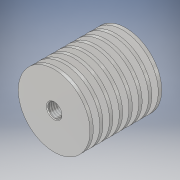
# Autodesk Inventor part: Cooling fin
Saved by Autodesk Inventor 2019 (Build 230136000, 136)
## iProperties
Created: 2018-11-13
Part Number: Cooling fin
Material: Aluminum 5005-H18
Document SubType Name: Modeling
Designer: LillaHunden
Density: 2.7 g/cm^3
Appearance: Aluminum - Polished
Author: LillaHunden
Autodesk Inventor part; units mm, degrees
ref_plane "YZ Plane" through (0, 0, 0) normal (1, 0, 0) x (0, 1, 0)
ref_plane "XZ Plane" through (0, 0, 0) normal (0, 1, 0) x (-1, 0, 0)
ref_plane "XY Plane" through (0, 0, 0) normal (0, 0, 1) x (1, 0, 0)
sketch "Sketch1" plane through (0, 0, 0) normal (0, 0, 1) x (1, 0, 0)
  circle A0 centre (0, 0) radius 12.5
  dimension "d0" = 25
  constraints: 1 centre point, 1 coincident
  measures "d0" diameter of A0
extrude "Extrusion1" add sketch "Sketch1" along normal blind 25
sketch "Sketch2" plane through (0, 0, 0) normal (1, 0, 0) x (0, 1, 0)
  line L0 (0, 0) -> (0, 24.8569) construction
  line L1 (12.5, 0) -> (12.5, 25) projected
  line L2 (12.5, 23.85) -> (4.58, 23.85)
  line L3 (4.58, 23.85) -> (4.58, 21.6)
  line L4 (4.58, 21.6) -> (12.5, 21.6)
  line L5 (12.5, 21.6) -> (12.5, 23.85)
  line L6 (12.5, 25) -> (-12.5, 25) projected
  line L7 (12.5, 20.45) -> (4.58, 20.45)
  line L8 (4.58, 20.45) -> (4.58, 18.2)
  line L9 (4.58, 18.2) -> (12.5, 18.2)
  line L10 (12.5, 18.2) -> (12.5, 20.45)
  line L11 (12.5, 17.05) -> (4.58, 17.05)
  line L12 (4.58, 17.05) -> (4.58, 14.8)
  line L13 (4.58, 14.8) -> (12.5, 14.8)
  line L14 (12.5, 14.8) -> (12.5, 17.05)
  line L15 (12.5, 13.65) -> (4.58, 13.65)
  line L16 (4.58, 13.65) -> (4.58, 11.4)
  line L17 (4.58, 11.4) -> (12.5, 11.4)
  line L18 (12.5, 11.4) -> (12.5, 13.65)
  line L19 (12.5, 10.25) -> (4.58, 10.25)
  line L20 (4.58, 10.25) -> (4.58, 8)
  line L21 (4.58, 8) -> (12.5, 8)
  line L22 (12.5, 8) -> (12.5, 10.25)
  line L23 (12.5, 6.85) -> (4.58, 6.85)
  line L24 (4.58, 6.85) -> (4.58, 4.6)
  line L25 (4.58, 4.6) -> (12.5, 4.6)
  line L26 (12.5, 4.6) -> (12.5, 6.85)
  line L27 (12.5, 3.45) -> (4.58, 3.45)
  line L28 (4.58, 3.45) -> (4.58, 1.2)
  line L29 (4.58, 1.2) -> (12.5, 1.2)
  line L30 (12.5, 1.2) -> (12.5, 3.45)
  dimension "d3" = 2.25
  dimension "d4" = 1.15
  dimension "d5" = 7.92
  dimension "d8" = 3.4
  constraints: 58 end point, 2 parallel, 2 vertical, 1 horizontal, 1 perpendicular, 1 point on line, 48 other
  measures "d3" distance of L2.end L3.end
  measures "d4" distance between parallel lines of L6 L2
  measures "d5" distance of L3.end L4.end
  measures "d8" distance of L2.start L7.start
revolve "Revolution1" cut sketch "Sketch2" angle 360 about axis through (0, 0, 0) along (0, 0, 1)
sketch "Sketch3" plane through (0, 0, 25) normal (0, 0, 1) x (1, 0, 0)
  circle A0 centre (0, 0) radius 2.46
  dimension "d14" = 4.92
  constraints: 1 centre point, 1 coincident
  measures "d14" diameter of A0
extrude "Extrusion2" cut sketch "Sketch3" against normal through all
thread "Thread1" size "M5x0.8" class "6H" standard "ANSI Metric M Profile" full length
chamfer "Chamfer1" distance 0.25 angle 45 1 edges at (-2.46, 0, 25)
chamfer "Chamfer2" distance 0.25 angle 45 1 edges at (-2.46, 0, 0)
body "Solid1"
